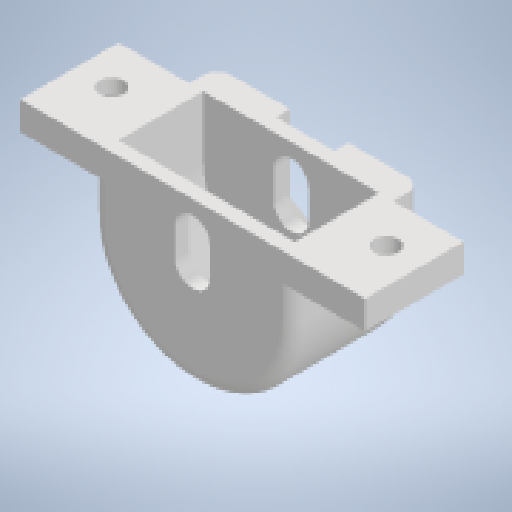
# Autodesk Inventor part: bearing_holder
Saved by Autodesk Inventor 2024 (Build 280153000, 153)
## iProperties
Created: 2026-02-05
Part Number: bearing_holder
Material: Generic
Document SubType Name: Modeling
Designer: SEMEN
Density: 1 g/cm^3
Appearance: Default
Author: SEMEN
Autodesk Inventor part; units mm, degrees
ref_plane "YZ Plane" through (0, 0, 0) normal (1, 0, 0) x (0, 1, 0)
ref_plane "XZ Plane" through (0, 0, 0) normal (0, 1, 0) x (-1, 0, 0)
ref_plane "XY Plane" through (0, 0, 0) normal (0, 0, 1) x (1, 0, 0)
sketch "Sketch1" plane through (0, 0, 0) normal (0, 0, 1) x (1, 0, 0)
  line L0 (25, 0) -> (25, 4) projected
  line L1 (0, 4) -> (25, 4) projected
  line L2 (0, 0) -> (0, 4) projected
  line L3 (16.65, -10.896) -> (12.5, -13.292)
  line L4 (12.5, -13.292) -> (8.35, -10.896)
  line L5 (8.35, -10.896) -> (8.35, -6.104)
  line L6 (16.65, -6.104) -> (16.65, -10.896)
  line L7 (8.35, -6.104) -> (8.35, 0)
  line L8 (16.65, -6.104) -> (16.65, 0)
  line L9 (25, -8.5) -> (25, 0)
  line L10 (0, -8.5) -> (0, 0)
  arc A0 (0, -8.5) -> (25, -8.5) centre (12.5, -8.5) ccw
  line L11 (10, -4.5) -> (10, -8.5)
  line L12 (15, -8.5) -> (15, -4.5)
  arc A1 (15, -4.5) -> (10, -4.5) centre (12.5, -4.5) ccw
  arc A2 (10, -8.5) -> (15, -8.5) centre (12.5, -8.5) ccw
  line L13 (-2, 0) -> (-2, -8.5)
  arc A3 (-2, -8.5) -> (27, -8.5) centre (12.5, -8.5) ccw
  line L14 (27, -8.5) -> (27, 0)
  line L15 (0, 0) -> (-2, 0)
  line L16 (-2, 0) -> (-5.3, 0)
  line L17 (-2, -4) -> (-12, -4)
  line L18 (-12, -4) -> (-12, 0)
  line L19 (-12, 0) -> (-8.7, 0)
  line L20 (27, -4) -> (37, -4)
  line L21 (37, -4) -> (37, 0)
  line L22 (37, 0) -> (33.7, 0)
  line L23 (25, 0) -> (27, 0)
  line L24 (27, 0) -> (30.3, 0)
  line L25 (25, 0) -> (16.65, 0)
  line L26 (8.35, 0) -> (16.65, 0)
  line L27 (8.35, 0) -> (0, 0)
  line L28 (33.7, 0) -> (30.3, 0) projected
  line L29 (-5.3, 0) -> (-8.7, 0) projected
  line L30 (32, 0) -> (32, -6.5) construction
  line L31 (-7, 0) -> (-7, -7.118) construction
  dimension "d5" = 8.3
  dimension "d7" = 5
  dimension "d8" = 2
  dimension "d9" = 4
  dimension "d10" = 4
  dimension "d13" = 8.5
  dimension "d14" = 12.5
  constraints: 54 end point, 8 point on circle, 6 perpendicular, 6 tangent, 4 centre point, 4 horizontal, 4 parallel, 4 point on line, 3 collinear, 2 midpoint, 2 symmetric about line, 2 vertical, 1 coincident, 10 other
  measures "d5" distance between parallel lines of L6 L5
  measures "d7" diameter of A2
  measures "d8" distance between parallel lines of L10 L13
  measures "d9" distance of L17.end L18.end
  measures "d10" distance of L20.end L21.end
  measures "d13" distance from line of L1 A1.centre
  measures "d14" distance from line of L1 point (12.5, -8.5)
extrude "Extrusion1" add sketch "Sketch1" along normal blind 12 contours L23 L14 A3 L13 L15 L10 A0 L9 | L24 L28 L22 L21 L20 L14 | L13 L17 L18 L19 L29 L16
sketch "Sketch2" plane through (0, 0, 0) normal (0, 0, -1) x (-1, 0, 0)
  line L0 (-25, 0) -> (-25, -8.5) projected
  arc A0 (-25, -8.5) -> (0, -8.5) centre (-12.5, -8.5) ccw projected
  line L1 (0, -8.5) -> (0, 0) projected
  line L2 (-27, -8.5) -> (-27, 0) projected
  arc A1 (-27, -8.5) -> (2, -8.5) centre (-12.5, -8.5) ccw projected
  line L3 (2, 0) -> (2, -8.5) projected
  line L4 (-8.35, -6.104) -> (-8.35, 0) projected
  line L5 (-8.35, -10.896) -> (-8.35, -6.104) projected
  line L6 (-12.5, -13.292) -> (-8.35, -10.896) projected
  line L7 (-16.65, -10.896) -> (-12.5, -13.292) projected
  line L8 (-16.65, -6.104) -> (-16.65, -10.896) projected
  line L9 (-16.65, -6.104) -> (-16.65, 0) projected
  line L10 (-15, -8.5) -> (-15, -4.5) projected
  arc A2 (-10, -4.5) -> (-15, -4.5) centre (-12.5, -4.5) ccw projected
  line L11 (-10, -4.5) -> (-10, -8.5) projected
  arc A3 (-15, -8.5) -> (-10, -8.5) centre (-12.5, -8.5) ccw projected
  line L12 (-245.5, 0) -> (14.5, 0) projected
extrude "Extrusion2" add sketch "Sketch2" along normal blind 4 contours L12 L9 L8 L7 L6 L5 L4 L1 A0 L0 | L0 A0 L1 L12 L3 A1 L2
sketch "Sketch3" plane through (0, 0, 0) normal (0, 0, 1) x (1, 0, 0)
  line L0 (8.35, 0) -> (8.35, -10.896) projected
  line L1 (12.5, -13.292) -> (8.35, -10.896) projected
  line L2 (12.5, -13.292) -> (16.65, -10.896) projected
  line L3 (16.65, -10.896) -> (16.65, 0) projected
  line L4 (15, -8.5) -> (15, -4.5) projected
  arc A0 (10, -8.5) -> (15, -8.5) centre (12.5, -8.5) ccw projected
  line L5 (10, -4.5) -> (10, -8.5) projected
  arc A1 (15, -4.5) -> (10, -4.5) centre (12.5, -4.5) ccw projected
  line L6 (92, 0) -> (245.5, 0) projected
  line L7 (245.5, 0) -> (-14.5, 0) projected
  point P0 (0, 0)
extrude "Extrusion3" add sketch "Sketch3" against normal blind 2
sketch "Sketch4" plane through (0, 0, 12) normal (0, 0, 1) x (1, 0, 0)
  arc A0 (15, -4.5) -> (10, -4.5) centre (12.5, -4.5) ccw projected
  line L0 (10, -8.5) -> (10, -4.5) projected
  arc A1 (10, -8.5) -> (15, -8.5) centre (12.5, -8.5) ccw projected
  line L1 (15, -4.5) -> (15, -8.5) projected
  line L2 (25, 0) -> (25, -8.5) projected
  arc A2 (0, -8.5) -> (25, -8.5) centre (12.5, -8.5) ccw projected
  line L3 (0, -8.5) -> (0, 0) projected
  line L4 (0, 0) -> (-12, 0) projected
  line L5 (-12, 0) -> (-12, -4) projected
  line L6 (-12, -4) -> (-2, -4) projected
  line L7 (-2, -4) -> (-2, -8.5) projected
  arc A3 (-2, -8.5) -> (27, -8.5) centre (12.5, -8.5) ccw projected
  line L8 (27, -8.5) -> (27, -4) projected
  line L9 (27, -4) -> (37, -4) projected
  line L10 (37, -4) -> (37, 0) projected
  line L11 (37, 0) -> (25, 0) projected
  line L12 (25, 0) -> (0, 0) projected
  line L13 (-2, -8.5) -> (-2, -4) projected
  line L14 (-2, -4) -> (-2, 0)
  line L15 (27, 0) -> (27, -8.5) projected
  line L16 (27, -4) -> (27, 0)
  constraints: 4 end point, 2 collinear
extrude "Extrusion4" add sketch "Sketch4" along normal blind 2
fillet "Fillet1" radius 2 6 edges at (27, -6.25, 14) (-2, -6.25, 14) (12.5, -23, 14) (-2, -4.25, -4) (27, -4.25, -4) (12.5, -23, -4)
sketch "Sketch5" plane through (27, -4, 0) normal (0, -1, 0) x (1, 0, 0)
  line L0 (7.85, 7.6454) -> (7.85, 4.3546)
  line L1 (7.85, 4.3546) -> (5, 2.7091)
  line L2 (5, 2.7091) -> (2.15, 4.3546)
  line L3 (2.15, 4.3546) -> (2.15, 7.6454)
  line L4 (2.15, 7.6454) -> (5, 9.2909)
  line L5 (5, 9.2909) -> (7.85, 7.6454)
  line L6 (-31.15, 7.6454) -> (-31.15, 4.3546)
  line L7 (-31.15, 4.3546) -> (-34, 2.7091)
  line L8 (-34, 2.7091) -> (-36.85, 4.3546)
  line L9 (-36.85, 4.3546) -> (-36.85, 7.6454)
  line L10 (-36.85, 7.6454) -> (-34, 9.2909)
  line L11 (-34, 9.2909) -> (-31.15, 7.6454)
  line L12 (10, 0) -> (10, 14) projected
  line L13 (-39, 0) -> (-39, 14) projected
  circle A0 centre (5, 6) radius 1.7
  circle A1 centre (-34, 6) radius 1.7
  point P0 (-27, 0)
  point P1 (10, 12)
  point P2 (-39, 12)
  dimension "d22" = 5.7
  dimension "d23" = 5.7
  constraints: 24 end point, 4 coincident, 2 centre point, 2 parallel, 30 other
  measures "d22" distance between parallel lines of L3 L0
  measures "d23" distance between parallel lines of L6 L9
extrude "Extrusion5" cut sketch "Sketch5" against normal blind 2 contours L0 L1 L2 L3 L4 L5 | L6 L7 L8 L9 L10 L11 | A0 | A1
hole "Hole1" at (32, -4, 6) at (-7, -4, 6) direction (0, 1, 0) diameter 3.4 end through all clearance for "Hex Head Bolt / Nut GOST 12876-67" size "M3" standard "GOST"
body "Solid1"
